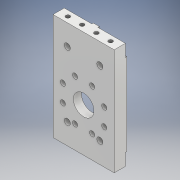
# Autodesk Inventor part: new_base_u64
Saved by Autodesk Inventor 2018 (Build 220112000, 112)
## iProperties
Created: 2016-12-19
Part Number: new_base_u64
Material: Aluminum 2014-T4
Document SubType Name: Modeling
Designer: steve
Density: 2.8 g/cm^3
Appearance: Satin
Mass: 18.4367 g
Surface Area: 50.621 cm^2
Volume: 6.58453 cm^3
Vendor: Rhoban
Author: steve
Autodesk Inventor part; units mm, degrees
ref_plane "YZ Plane" through (0, 0, 0) normal (1, 0, 0) x (0, 1, 0)
ref_plane "XZ Plane" through (0, 0, 0) normal (0, 1, 0) x (-1, 0, 0)
ref_plane "XY Plane" through (0, 0, 0) normal (0, 0, 1) x (1, 0, 0)
sketch "Sketch1" plane through (0, 0, 0) normal (0, 1, 0) x (-1, 0, 0)
  line L0 (15, 30.94) -> (-15, 30.94)
  line L1 (-15, 30.94) -> (-15, -21.4)
  line L2 (-15, -21.4) -> (15, -21.4)
  line L3 (15, -21.4) -> (15, 30.94)
  line L4 (0, 30.94) -> (0, -21.4) construction
  line L5 (15, 0) -> (-15, 0) construction
  line L6 (15, 4.77) -> (-15, 4.77) construction
  point P0 (0, 0)
  point P1 (0, 0)
  dimension "d0" = 52.34
  dimension "d1" = 30
  dimension "d64" = 4.77
  constraints: 14 end point, 5 midpoint, 2 parallel, 2 perpendicular, 2 point on line, 1 coincident, 1 horizontal
  measures "d0" distance of L2.end L0.start
  measures "d1" distance between parallel lines of L1 L3
  measures "d64" distance between parallel lines of L5 L6
extrude "Extrusion1" add sketch "Sketch1" along normal blind 6.25
sketch "Sketch2" plane through (0, 6.25, 0) normal (0, 1, 0) x (1, 0, 0)
  circle A0 centre (0, 0) radius 11 construction
  line L0 (0, 0) -> (-4.2095, -10.1627) construction
  line L1 (-15, -30.94) -> (15, -30.94) projected
  line L2 (15, -30.94) -> (15, 21.4) projected
  line L3 (15, 21.4) -> (-15, 21.4) projected
  line L4 (-15, 21.4) -> (-15, -30.94) projected
  line L5 (0, 0) -> (-4.2095, -10.1627) construction
  line L6 (0, 0) -> (0, -30.94) construction
  point P0 (4.2095, -10.1627)
  point P1 (10.1627, -4.2095)
  point P2 (10.1627, 4.2095)
  point P3 (4.2095, 10.1627)
  point P4 (-4.2095, 10.1627)
  point P5 (-10.1627, 4.2095)
  point P6 (-10.1627, -4.2095)
  dimension "d7" = 22
  dimension "d8" = 360
  dimension "d98" = 22.5
  constraints: 6 end point, 3 coincident, 3 point on circle, 1 centre point, 1 midpoint, 1 point on line, 9 other
  measures "d7" diameter of A0
  measures "d98" angle of L6 L5
hole "Hole1" at (-4.2095, 6.25, 10.1627) at (-10.1627, 6.25, 4.2095) at (-10.1627, 6.25, -4.2095) at (-4.2095, 6.25, -10.1627) at (4.2095, 6.25, -10.1627) at (10.1627, 6.25, -4.2095) at (10.1627, 6.25, 4.2095) at (4.2095, 6.25, 10.1627) direction (0, -1, 0) diameter 2.5 end through all
sketch "Sketch3" plane through (0, 6.25, 0) normal (0, 1, 0) x (1, 0, 0)
  circle A0 centre (0, 0) radius 5.05
  dimension "d17" = 10.1
  constraints: 1 centre point, 1 coincident
  measures "d17" diameter of A0
extrude "Extrusion2" cut sketch "Sketch3" against normal through all
sketch "Sketch4" plane through (0, 6.25, 0) normal (0, 1, 0) x (1, 0, 0)
  line L0 (-8, -20.77) -> (8, -20.77) construction
  line L1 (8, -20.77) -> (8, 11.23) construction
  line L2 (8, 11.23) -> (-8, 11.23) construction
  line L3 (-8, 11.23) -> (-8, -20.77) construction
  line L4 (-15, -30.94) -> (15, -30.94) construction
  line L5 (0, -30.94) -> (0, 21.4) construction
  line L6 (15, 21.4) -> (-15, 21.4) construction
  line L7 (-15, 21.4) -> (-15, -30.94) construction
  line L8 (-15, -4.77) -> (15, -4.77) construction
  line L9 (15, -30.94) -> (15, 21.4) construction
  line L10 (0, -20.77) -> (0, 11.23) construction
  line L11 (-8, -4.77) -> (8, -4.77) construction
  point P0 (0, 0)
  dimension "d20" = 32
  dimension "d21" = 16
  constraints: 16 end point, 8 midpoint, 4 coincident, 2 collinear, 2 parallel, 1 horizontal, 1 perpendicular
  measures "d20" distance of L2.end L0.start
  measures "d21" distance of L1.end L2.end
hole "Hole2" at (-8, 6.25, 20.77) at (8, 6.25, 20.77) at (8, 6.25, -11.23) at (-8, 6.25, -11.23) direction (0, -1, 0) diameter 3 end through all
sketch "Sketch6" plane through (-15, 0, 30.94) normal (0, 0, 1) x (1, 0, 0)
  line L0 (-10.3797, 2.75) -> (37.9037, 2.75) construction
  line L1 (0, 0) -> (30, 0) construction
  line L2 (0, 0) -> (0, 6.25) projected
  point P0 (15, 0)
  point P1 (4.5, 2.75)
  point P2 (11.5, 2.75)
  point P3 (18.5, 2.75)
  point P4 (25.5, 2.75)
  dimension "d33" = 2.75
  dimension "d34" = 4.5
  dimension "d37" = 7
  constraints: 2 end point, 2 horizontal, 1 point on line, 3 other
  measures "d33" distance between parallel lines of L1 L0
  measures "d34" distance from line of L2 point (4.5, 2.75)
  measures "d37" distance of point (4.5, 2.75) point (11.5, 2.75)
hole "Hole3" at (-10.5, 2.75, 30.94) at (-3.5, 2.75, 30.94) at (3.5, 2.75, 30.94) at (10.5, 2.75, 30.94) direction (0, 0, -1) diameter 2.013 depth 7.6 tip angle 118 thread size "M2.5x0.45" class "6H" standard "ANSI Metric M Profile"
sketch "Sketch7" plane through (15, 0, -21.4) normal (0, 0, -1) x (-1, 0, 0)
  line L0 (-10.51, 2.75) -> (37.7733, 2.75) construction
  line L1 (0, 0) -> (29.8697, 0) construction
  line L2 (0, 0) -> (0, 3.7534)
  line L3 (0, 0) -> (30, 0) projected
  line L4 (0, 0) -> (0, 6.25) projected
  point P0 (15, 0)
  point P1 (15, 0)
  point P2 (4.5, 2.75)
  point P3 (11.5, 2.75)
  point P4 (18.5, 2.75)
  point P5 (25.5, 2.75)
  dimension "d53" = 2.75
  dimension "d54" = 4.5
  dimension "d55" = 7
  constraints: 6 end point, 2 collinear, 2 horizontal, 1 point on line, 3 other
  measures "d53" distance between parallel lines of L1 L0
  measures "d54" distance from line of L2 point (4.5, 2.75)
  measures "d55" distance of point (4.5, 2.75) point (11.5, 2.75)
hole "Hole4" at (10.5, 2.75, -21.4) at (-10.5, 2.75, -21.4) at (-3.5, 2.75, -21.4) at (3.5, 2.75, -21.4) direction (0, 0, 1) diameter 2.013 depth 7.6 tip angle 118 thread size "M2.5x0.45" class "6H" standard "ANSI Metric M Profile"
sketch "Sketch8" plane through (0, 6.25, 0) normal (0, 1, 0) x (1, 0, 0)
  line L0 (0, 32.012) -> (0, -41.432) construction
  line L1 (-15, -30.94) -> (15, -30.94) projected
  line L2 (15, 21.4) -> (-15, 21.4) projected
  line L3 (-1.5, -30.94) -> (-15, -30.94)
  line L4 (-15, -30.94) -> (-15, -24.94)
  line L5 (-15, -24.94) -> (-1.5, -24.94)
  line L6 (1.5, -30.94) -> (15, -30.94)
  line L7 (15, -30.94) -> (15, -24.94)
  line L8 (15, -24.94) -> (1.5, -24.94)
  line L9 (15, -30.94) -> (15, 21.4) projected
  line L10 (-15, 21.4) -> (-15, -30.94) projected
  line L11 (-1.5, -24.94) -> (-1.5, -30.94)
  line L12 (-15, -30.94) -> (15, -30.94) projected
  line L13 (1.5, -24.94) -> (1.5, -30.94)
  line L14 (-15, -4.77) -> (15, -4.77) construction
  line L15 (-1.5, 21.4) -> (-15, 21.4)
  line L16 (-15, 21.4) -> (-15, 15.4)
  line L17 (-15, 15.4) -> (-1.5, 15.4)
  line L18 (1.5, 21.4) -> (15, 21.4)
  line L19 (15, 21.4) -> (15, 15.4)
  line L20 (15, 15.4) -> (1.5, 15.4)
  line L21 (-1.5, 15.4) -> (-1.5, 21.4)
  line L22 (1.5, 15.4) -> (1.5, 21.4)
  line L23 (-21.8515, -28.94) -> (23.2072, -28.94) construction
  point P0 (0, 0)
  dimension "d80" = 6
  dimension "d81" = 3
  dimension "d82" = 13.5
  dimension "d86" = 2
  constraints: 36 end point, 7 symmetric about line, 4 point on line, 3 collinear, 3 horizontal, 3 parallel, 3 perpendicular, 2 midpoint
  measures "d80" distance between parallel lines of L1 L5
  measures "d81" distance between parallel lines of L13 L11
  measures "d82" distance between parallel lines of L7 L13
  measures "d86" distance between parallel lines of L1 L23
sketch "Sketch9" plane through (0, 6.25, 0) normal (0, 1, 0) x (1, 0, 0)
  circle A0 centre (-4.2095, -10.1627) radius 1.25 construction
  circle A1 centre (4.2095, -10.1627) radius 1.25 construction
  circle A2 centre (10.1627, -4.2095) radius 1.25 construction
  circle A3 centre (10.1627, 4.2095) radius 1.25 construction
  circle A4 centre (4.2095, 10.1627) radius 1.25 construction
  circle A5 centre (-4.2095, 10.1627) radius 1.25 construction
  circle A6 centre (-10.1627, 4.2095) radius 1.25 construction
  circle A7 centre (-10.1627, -4.2095) radius 1.25 construction
  circle A8 centre (0, 0) radius 11 construction
  constraints: 1 coincident, 3 other
hole "Hole5" at (-4.2095, 6.25, 10.1627) at (4.2095, 6.25, 10.1627) at (10.1627, 6.25, 4.2095) at (10.1627, 6.25, -4.2095) at (4.2095, 6.25, -10.1627) at (-4.2095, 6.25, -10.1627) at (-10.1627, 6.25, -4.2095) at (-10.1627, 6.25, 4.2095) direction (0, -1, 0) diameter 5 depth 2.175
extrude "Extrusion6" cut sketch "Sketch8" against normal blind 0.75 contours L4 L5 L11 L1 | L13 L8 L7 L1 | L10 L2 L21 L17 | L20 L22 L2 L9
fillet "Fillet1" radius 3 4 edges at (1.5, 5.875, 24.94) (-1.5, 5.875, 24.94) (1.5, 5.875, -15.4) (-1.5, 5.875, -15.4)
sketch "Sketch11" plane through (0, 6.25, 0) normal (0, 1, 0) x (1, 0, 0)
  line L0 (-13.5, -23.44) -> (13.5, -23.44)
  line L1 (13.5, -23.44) -> (13.5, 13.9)
  line L2 (13.5, 13.9) -> (-13.5, 13.9)
  line L3 (-13.5, 13.9) -> (-13.5, -23.44)
  line L4 (-15, 15.4) -> (-15, -24.94) projected
  line L5 (15, -24.94) -> (15, 15.4) projected
  line L6 (-1.5, -30.94) -> (-15, -30.94) projected
  line L7 (-15, 21.4) -> (-1.5, 21.4) projected
  circle A0 centre (-8, 11.23) radius 3 construction
  arc A1 (-6.5016, 11.1609) -> (-6.6857, 10.5071) centre (-8, 11.23) ccw construction
  point P0 (0, 0)
  dimension "d87" = 7.5
  dimension "d88" = 7.5
  dimension "d91" = 1.5
  dimension "d92" = 1.5
  dimension "d93" = 6
  constraints: 8 end point, 2 parallel, 1 centre point, 1 concentric, 1 horizontal, 1 perpendicular
  measures "d87" distance between parallel lines of L6 L0
  measures "d88" distance between parallel lines of L7 L2
  measures "d91" distance between parallel lines of L4 L3
  measures "d92" distance between parallel lines of L5 L1
  measures "d93" diameter of A0
extrude "Extrusion7" cut sketch "Sketch11" against normal blind 2.25
fillet "Fillet2" radius 1.5 4 edges at (-13.5, 5.125, 23.44) (13.5, 5.125, 23.44) (13.5, 5.125, -13.9) (-13.5, 5.125, -13.9)
equation "\"d0\" = total_width"
equation "\"d64\" = axis_offset"
equation "\"d3\" = plate_thickness"
equation "\"d7\" = d9"
equation "\"d18\" = plate_thickness"
equation "\"d33\" = hole_2_bottom"
equation "\"d53\" = hole_2_bottom"
equation "\"d83\" = plate_thickness - border_thickness"
equation "\"plate_thickness\" = 6.25"
equation "\"d9\" = 22"
equation "\"tol\" = 0.1"
equation "\"border_thickness\" = 5.5"
equation "\"hole_2_bottom\" = 0.5 * border_thickness"
equation "\"central_thickness\" = 4"
equation "\"side_thickness\" = 3"
equation "\"side_trace_depth\" = 1"
equation "\"internal_width\" = bloc_106_spacing - side_thickness"
equation "\"total_width\" = internal_width + 2 * side_trace_depth"
equation "\"axis_offset\" = 0.5 * internal_width + side_thickness - axis_to_N102"
equation "\"bloc_106_spacing\" = 53.34"
equation "\"axis_to_N102\" = 23.4"
body "Solid1"
